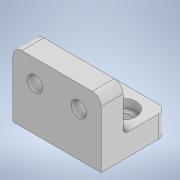
# Autodesk Inventor part: Brackets RC mounting board
Saved by Autodesk Inventor 2020.4 (Build 244396000, 396)
## iProperties
Created: 2021-05-03
Part Number: Brackets RC mounting board
Material: Generic
Document SubType Name: Modeling
Designer: Brandon
Density: 1 g/cm^3
Appearance: Default
Author: Brandon
Autodesk Inventor part; units mm, degrees
ref_plane "YZ Plane" through (0, 0, 0) normal (1, 0, 0) x (0, 1, 0)
ref_plane "XZ Plane" through (0, 0, 0) normal (0, 1, 0) x (-1, 0, 0)
ref_plane "XY Plane" through (0, 0, 0) normal (0, 0, 1) x (1, 0, 0)
sketch "Sketch1" plane through (0, 0, 0) normal (0, 1, 0) x (-1, 0, 0)
  line L0 (10, 0) -> (-10, 0)
  line L1 (10, -5) -> (-10, -5)
  line L2 (-10, 0) -> (-10, -15)
  line L3 (-10, -15) -> (10, -15)
  line L4 (10, -15) -> (10, 0)
  point P0 (0, 0)
  dimension "d15" = 15
  dimension "d16" = 20
  constraints: 10 end point, 2 perpendicular, 1 vertical
  measures "d15" distance of L0.end L2.end
  measures "d16" distance of L2.end L3.end
extrude "Extrusion1" add sketch "Sketch1" along normal blind 15 contours L4 L1 L2 L0
extrude "Extrusion2" add sketch "Sketch1" along normal blind 5 contours L4 L3 L2 L1
sketch "Sketch2" plane through (0, 5, 0) normal (0, 1, 0) x (1, 0, 0)
  line L0 (-10, 15) -> (-10, 0) projected
  line L1 (-10, 15) -> (-5, 15)
  line L2 (10, 15) -> (-10, 15) projected
  line L3 (-5, 15) -> (-5, 10)
  line L4 (10, 15) -> (5, 15)
  line L5 (5, 15) -> (5, 10)
  point P0 (0, 0)
  dimension "d21" = 5
  dimension "d22" = 5
  dimension "d23" = 5
  dimension "d24" = 5
  dimension "d60" = 10
  constraints: 8 end point, 2 point on line, 1 perpendicular, 1 vertical
  measures "d21" distance of L0.start L1.end
  measures "d22" distance of L1.end L3.end
  measures "d23" distance of L4.start L4.end
  measures "d24" distance of L4.end L5.end
  measures "d60" distance between parallel lines of L5 L3
hole "Hole1" at (-5, 5, -10) direction (0, -1, 0) diameter 3.5 end through all counterbore diameter 6 counterbore depth 2
hole "Hole2" at (5, 5, -10) direction (0, -1, 0) diameter 3.5 end through all counterbore diameter 6 counterbore depth 2
sketch "Sketch3" plane through (10, 15, -5) normal (0, 0, -1) x (-1, 0, 0)
  line L0 (20, -10) -> (20, 0) projected
  line L1 (20, 0) -> (15, 0)
  line L2 (0, 0) -> (20, 0) projected
  line L3 (15, 0) -> (15, -5)
  line L4 (0, -10) -> (0, 0) projected
  line L5 (0, 0) -> (5, 0)
  line L6 (5, 0) -> (5, -5)
  point P0 (10, -15)
  dimension "d39" = 5
  dimension "d40" = 5
  dimension "d41" = 5
  dimension "d42" = 5
  constraints: 8 end point, 2 point on line, 1 perpendicular, 1 vertical
  measures "d39" distance of L0.end L1.end
  measures "d40" distance of L1.end L3.end
  measures "d41" distance of L2.start L5.end
  measures "d42" distance of L5.end L6.end
hole "Hole3" at (-5, 10, -5) direction (0, 0, 1) diameter 3.5 end through all counterbore diameter 6 counterbore depth 2
hole "Hole4" at (5, 10, -5) direction (0, 0, 1) diameter 3.5 end through all counterbore diameter 6 counterbore depth 2
fillet "Fillet2" radius 2 4 edges at (-10, 2.5, -15) (10, 2.5, -15) (10, 15, -2.5) (-10, 15, -2.5)
fillet "Fillet2" radius 1 1 edges at (0, 5, -5)
body "Solid1"
